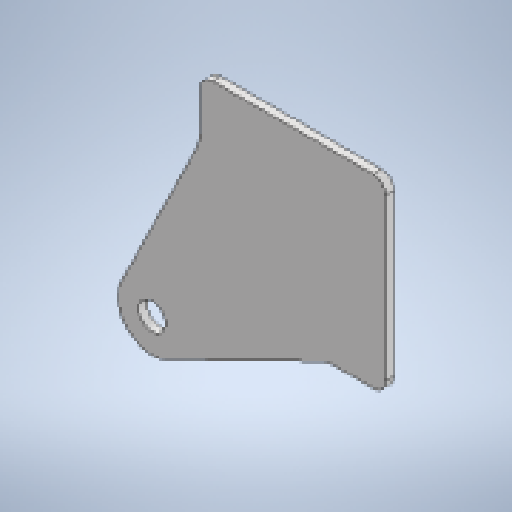
# Autodesk Inventor part: MSC 128 base plate
Saved by Autodesk Inventor 2025 (Build 290162010, 162A)
## iProperties
Created: 2024-07-01
Part Number: MSC 128 base plate
Material: Stainless Steel
Document SubType Name: Sheet Metal
Designer: admin
Density: 8 g/cm^3
Sheet Metal Rule: AISI304 4mm Die 32
Appearance: Default
Flat Pattern Width: 11.6404 cm
Flat Pattern Length: 16.6102 cm
Flat Pattern Area: 193.35 cm^2
Sheet Metal Width: 116,404 mm
Sheet Metal Length: 166,102 mm
Sheet Metal Area: 19334,975 mm^2
Author: pokla
Autodesk Inventor part; units mm, degrees
ref_plane "YZ Plane" through (0, 0, 0) normal (1, 0, 0) x (0, 1, 0)
ref_plane "XZ Plane" through (0, 0, 0) normal (0, 1, 0) x (-1, 0, 0)
ref_plane "XY Plane" through (0, 0, 0) normal (0, 0, 1) x (1, 0, 0)
sketch "Sketch1" plane through (0, 0, 0) normal (0, 1, 0) x (-1, 0, 0)
  line L0 (40, 40) -> (-40, 40) construction
  line L1 (-40, 40) -> (-40, -40) construction
  line L2 (-40, -40) -> (40, -40) construction
  line L3 (40, -40) -> (40, 40) construction
  line L4 (-40, 40) -> (40, -40) construction
  line L5 (0, 40) -> (0, -40) construction
  line L6 (-45, -45) -> (-45, 0)
  line L7 (-20, -45) -> (-45, -45)
  arc A0 (61.0074, -83.093) -> (83.093, -61.0074) centre (68.2843, -68.2843) ccw
  circle A1 centre (68.2843, -68.2843) radius 6.5
  line L8 (61.0074, -83.093) -> (-13.3847, -46.5375)
  arc A2 (-13.3847, -46.5375) -> (-20, -45) centre (-20, -60) ccw
  arc A3 (83.093, -61.0074) -> (61.0074, -83.093) centre (68.2843, -68.2843) ccw construction
  line L9 (83.093, -61.0074) -> (46.5375, 13.3847)
  line L10 (-45, 0) -> (-45, 45)
  line L11 (-45, 45) -> (45, 45)
  line L12 (45, 45) -> (45, 20)
  arc A4 (45, 20) -> (46.5375, 13.3847) centre (60, 20) ccw
  line L13 (40, 0) -> (45, 0) construction
  line L14 (0, 40) -> (0, 45) construction
  line L15 (-40, 0) -> (-45, 0) construction
  point P0 (0, 0)
  point P1 (0, 0)
  point P2 (0, 0)
  dimension "d2" = 80
  dimension "d3" = 80
  dimension "d29" = 5
  dimension "d30" = 13
  dimension "d31" = 10
  dimension "d32" = 40
  dimension "d34" = 5
  dimension "d35" = 15
  dimension "d36" = 25
  measures "d2" distance of L2.end L1.end
  measures "d3" distance of L1.end L0.end
  measures "d29" distance between parallel lines of L6 L1
  measures "d30" diameter of A1
  measures "d31" radial gap between concentric circles of A0 A1
  measures "d32" distance of L2.end A1.centre
  measures "d34" distance between parallel lines of L2 L7
  measures "d35" radius of A2
  measures "d36" distance of L7.start L6.start
extrude "Plate1" add sketch "Sketch1" along normal blind 4
fillet "Corner Round3" radius 6 3 edges at (-45, 2, 45) (45, 2, 45) (45, 2, -45)
equation "\"d34\" = d29"
equation "\"d6\" = Thickness"
equation "\"Thickness\" = 4"
body "Solid1"
